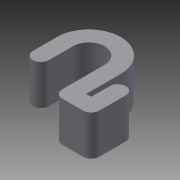
# Autodesk Inventor part: Percha
Saved by Autodesk Inventor 2014 (Build 180170000, 170)
## iProperties
Created: 2015-04-07
Part Number: Percha
Material: Generic
Document SubType Name: Modeling
Designer: Rubén
Density: 1 g/cm^3
Appearance: Default
Author: Rubén
Autodesk Inventor part; units mm, degrees
ref_plane "YZ Plane" through (0, 0, 0) normal (1, 0, 0) x (0, 1, 0)
ref_plane "XZ Plane" through (0, 0, 0) normal (0, 1, 0) x (-1, 0, 0)
ref_plane "XY Plane" through (0, 0, 0) normal (0, 0, 1) x (1, 0, 0)
sketch "Sketch1" plane through (0, 0, 0) normal (0, 1, 0) x (-1, 0, 0)
  line L0 (0, 0) -> (-1.9, 0)
  line L1 (-1.9, 0) -> (-1.9, -7)
  line L2 (-4.9, -10) -> (-4.9, -10)
  line L3 (-7.9, -7) -> (-7.9, 3)
  line L4 (-4.9, 6) -> (3, 6)
  line L5 (0, 0) -> (0, -13)
  line L6 (12, -25) -> (12, -25)
  line L7 (24, -13) -> (24, -4)
  line L8 (21, -1) -> (21, -1)
  line L9 (18, -4) -> (18, -13)
  line L10 (12, -19) -> (12, -19)
  line L11 (6, -13) -> (6, 3)
  arc A0 (6, -13) -> (12, -19) centre (12, -13) ccw
  arc A1 (12, -19) -> (18, -13) centre (12, -13) ccw
  arc A2 (0, -13) -> (12, -25) centre (12, -13) ccw
  arc A3 (12, -25) -> (24, -13) centre (12, -13) ccw
  arc A4 (-4.9, 6) -> (-7.9, 3) centre (-4.9, 3) ccw
  arc A5 (6, 3) -> (3, 6) centre (3, 3) ccw
  arc A6 (-4.9, -10) -> (-1.9, -7) centre (-4.9, -7) ccw
  arc A7 (-7.9, -7) -> (-4.9, -10) centre (-4.9, -7) ccw
  arc A8 (24, -4) -> (21, -1) centre (21, -4) ccw
  arc A9 (21, -1) -> (18, -4) centre (21, -4) ccw
  point P0 (-1.9, -10)
  point P1 (-7.9, -10)
  point P2 (-7.9, 6)
  point P3 (6, 6)
  point P4 (0, -25)
  point P5 (24, -25)
  point P6 (24, -1)
  point P7 (18, -1)
  point P8 (18, -19)
  point P9 (6, -19)
  dimension "d0" = 1.9
  dimension "d1" = 10
  dimension "d2" = 6
  dimension "d3" = 16
  dimension "d4" = 6
  dimension "d5" = 25
  dimension "d6" = 24
  dimension "d7" = 24
  dimension "d8" = 6
  dimension "d9" = 18
  dimension "d10" = 12
  dimension "d11" = 6
  dimension "d12" = 12
  dimension "d13" = 3
  constraints: 24 end point, 20 point on circle, 20 point on line, 20 tangent, 10 centre point, 7 equal radius, 5 parallel, 5 perpendicular, 1 horizontal
  measures "d0" distance of L0.start L0.end
  measures "d1" distance of L0.end point (-1.9, -10)
  measures "d2" distance of point (-1.9, -10) point (-7.9, -10)
  measures "d3" distance of point (-7.9, -10) point (-7.9, 6)
  measures "d4" horizontal distance of L0.start point (6, 6)
  measures "d5" distance of L0.start point (0, -25)
  measures "d6" distance of point (0, -25) point (24, -25)
  measures "d7" distance of point (24, -25) point (24, -1)
  measures "d8" distance of point (24, -1) point (18, -1)
  measures "d9" distance of point (18, -1) point (18, -19)
  measures "d10" distance of point (18, -19) point (6, -19)
  measures "d11" radius of A0
  measures "d12" radius of A2
  measures "d13" radius of A4
extrude "Extrusion1" add sketch "Sketch1" along normal blind 15
body "Solid1"
